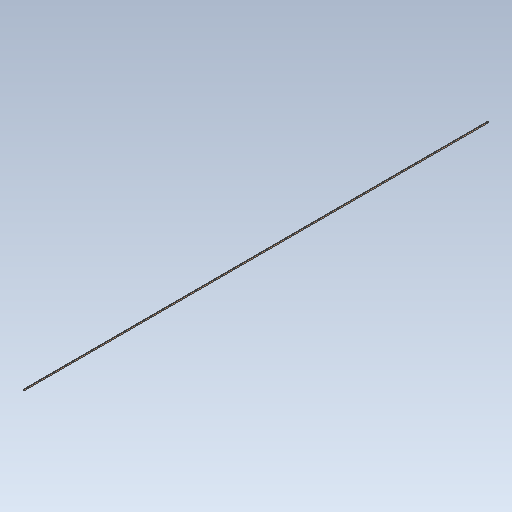
# Autodesk Inventor part: led-liste
Saved by Autodesk Inventor 2020.1 (Build 241239000, 239)
## iProperties
Created: 2021-09-24
Part Number: led-liste
Material: Wood (Birch)
Document SubType Name: Modeling
Designer: loppen
Density: 0.55 g/cm^3
Appearance: Birch - Natural Polished
Author: loppen
Autodesk Inventor part; units mm, degrees
ref_plane "YZ Plane" through (0, 0, 0) normal (1, 0, 0) x (0, 1, 0)
ref_plane "XZ Plane" through (0, 0, 0) normal (0, 1, 0) x (-1, 0, 0)
ref_plane "XY Plane" through (0, 0, 0) normal (0, 0, 1) x (1, 0, 0)
sketch "Sketch1" plane through (0, 0, 0) normal (0, 0, 1) x (1, 0, 0)
  line L0 (0, 0) -> (6, 0)
  line L1 (6, 0) -> (6, 12)
  line L2 (6, 12) -> (0, 12)
  line L3 (0, 12) -> (0, 0)
  dimension "d0" = 6
  dimension "d1" = 12
  constraints: 8 end point, 2 parallel, 1 horizontal, 1 perpendicular
  measures "d0" distance of L2.end L1.end
  measures "d1" distance of L1.end L0.end
extrude "Extrusion1" add sketch "Sketch1" along normal blind 4830.551
body "Solid1"
